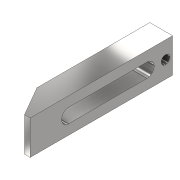
# Autodesk Inventor part: Lengueta 2 LRP
Saved by Autodesk Inventor 2020.3 (Build 243373000, 373)
## iProperties
Created: 2020-05-30
Part Number: Lengueta 2 LRP
Material: Steel, High Strength, Low Alloy
Document SubType Name: Modeling
Designer: Pipi
Density: 7.85 g/cm^3
Appearance: Steel - Polished
Author: Pipi
Autodesk Inventor part; units mm, degrees
ref_plane "YZ Plane" through (0, 0, 0) normal (1, 0, 0) x (0, 1, 0)
ref_plane "XZ Plane" through (0, 0, 0) normal (0, 1, 0) x (-1, 0, 0)
ref_plane "XY Plane" through (0, 0, 0) normal (0, 0, 1) x (1, 0, 0)
sketch "Boceto1" plane through (0, 0, 0) normal (0, 1, 0) x (-1, 0, 0)
  line L0 (3.0387, 27.5812) -> (3.0387, -22.4188)
  line L1 (3.0387, -22.4188) -> (11.0387, -22.4188)
  line L2 (11.0387, -22.4188) -> (11.0387, 17.1889)
  line L3 (3.0387, 27.5812) -> (5.0387, 27.5812)
  line L4 (5.0387, 27.5812) -> (11.0387, 17.1889)
  dimension "d0" = 50
  dimension "d1" = 8
  dimension "d3" = 2
  dimension "d69" = 30
  constraints: 10 end point, 2 perpendicular, 1 horizontal, 1 vertical
  measures "d0" distance of L0.start L0.end
  measures "d1" distance of L0.end L1.end
  measures "d3" distance of L0.start L3.end
  measures "d69" angle of L0 L4
extrude "Extrusión1" add sketch "Boceto1" along normal blind 12
sketch "Boceto3" plane through (-11.0387, 0, -22.4188) normal (-1, 0, 0) x (0, 0, 1)
  line L0 (0, 0) -> (0, 12) projected
  line L1 (39.6077, 0) -> (39.6077, 12) projected
  line L2 (0, 12) -> (39.6077, 12) projected
  circle A0 centre (2.5, 6) radius 1.5
  line L3 (9, 3.5) -> (36.5, 3.5)
  line L4 (9, 8.5) -> (36.5, 8.5)
  line L5 (0, 0) -> (39.6077, 0) projected
  arc A1 (9, 8.5) -> (9, 3.5) centre (9, 6) ccw
  circle A2 centre (9, 6) radius 4.5
  circle A3 centre (36.5, 6) radius 2.5
  dimension "d51" = 3
  dimension "d52" = 2.5
  dimension "d56" = 27.5
  dimension "d63" = 5
  dimension "d64" = 9
  dimension "d65" = 27.5
  dimension "d66" = 9
  constraints: 4 end point, 3 centre point, 2 horizontal, 2 point on circle, 1 coincident, 3 other
  measures "d51" diameter of A0
  measures "d52" distance from line of A0.centre L0
  measures "d56" distance of L4.start L4.end
  measures "d63" diameter of A1
  measures "d64" distance from line of A1.centre L0
  measures "d65" distance of L3.start L3.end
  measures "d66" diameter of A2
extrude "Extrusión6" cut sketch "Boceto3" against normal blind 10 contours A0 | A1 L4 A2 L3 | A2 L4 A3 L3 | A3 picked at (10.5, 6)
thread "Thread1" size "M3x0.5" class "6H" standard "ISO Metric profile" length 98
